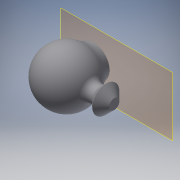
# Autodesk Inventor part: The Thing
Saved by Autodesk Inventor 2017 (Build 210142000, 142)
## iProperties
Created: 2017-03-09
Part Number: The Thing
Material: Generic
Document SubType Name: Modeling
Designer: PLTW
Density: 1 g/cm^3
Appearance: Default
Author: PLTW
Autodesk Inventor part; units mm, degrees
ref_plane "YZ Plane" through (0, 0, 0) normal (1, 0, 0) x (0, 1, 0)
ref_plane "XZ Plane" through (0, 0, 0) normal (0, 1, 0) x (-1, 0, 0)
sketch "Sketch3" plane through (0, 0, 0) normal (0, 0, 1) x (1, 0, 0)
  line L0 (-10.8841, 4.3559) -> (-10.16, 5.08)
  line L1 (-7.62, -2.54) -> (-10.16, -5.08)
  line L2 (-10.16, -5.08) -> (-10.8841, -4.3559)
  line L3 (-10.8912, 3.81) -> (-8.255, 6.4462)
  line L4 (-8.255, 6.4462) -> (-4.191, 2.3822)
  line L5 (-4.191, 2.3822) -> (-4.191, 0)
  line L6 (-4.191, 0) -> (-16.6062, 0)
  line L7 (-10.8912, 3.81) -> (-16.6062, 3.81)
  line L8 (-16.6062, 3.81) -> (-16.6062, 0)
  line L9 (-10.8841, 4.3559) -> (-9.525, 5.715)
  line L10 (-9.525, -5.715) -> (-10.8841, -4.3559)
  line L11 (-8.255, 6.985) -> (-3.81, 2.54)
  line L12 (-3.81, 2.54) -> (-3.81, -2.54)
  line L13 (-3.81, -2.54) -> (-8.255, -6.985)
  point P0 (0, 0)
  point P1 (-7.62, 0)
  dimension "d5" = 0.381
  dimension "d12" = 5.715
  dimension "d13" = 3.81
  dimension "d26" = 0.381
  dimension "d27" = 0.381
  constraints: 28 end point, 3 perpendicular, 2 horizontal alignment, 2 vertical, 1 horizontal, 1 parallel, 23 other
  measures "d5" distance between parallel lines of L0 L3
  measures "d12" distance of L3.start L7.end
  measures "d13" distance of L7.end L6.end
  measures "d26" distance between parallel lines of L11 L4
  measures "d27" distance between parallel lines of L12 L5
revolve "Revolution2" add sketch "Sketch3" angle 360 about axis through (-4.191, 0, 0) along (-1, 0, 0)
fillet "Fillet2" radius 0.127 3 edges at (-8.255, -6.4462, 0) (-10.8912, -3.81, 0) (-4.191, -2.3822, 0)
sketch "Sketch5" plane through (0, 0, 0) normal (0, 1, 0) x (-1, 0, 0)
  line L0 (16.6062, 3.81) -> (16.6062, -3.81) projected
  line L1 (16.6062, 3.81) -> (16.6062, -3.81) projected
  line L2 (10.9438, 3.81) -> (10.9438, -3.81) projected
  arc A0 (26.7662, 12.7) -> (26.7662, -12.7) centre (26.7662, 0) ccw
  line L3 (26.7662, 12.7) -> (26.7662, -12.7)
  point P0 (0, 0)
  dimension "d14" = 25.4
  dimension "d15" = 2.54
  constraints: 3 point on circle, 2 end point, 2 vertical alignment, 1 centre point, 1 horizontal alignment, 1 vertical
  measures "d14" distance of L3.end A0.start
  measures "d15" distance edge to line of A0 L0
revolve "Revolution3" add sketch "Sketch5" angle 360 about axis through (-26.7662, 0, 12.7) along (0, 0, -1)
ref_plane "Work Plane1" through (0, 0, -12.7) normal (0, 0, 1) x (1, 0, 0)
sketch "Sketch8" plane through (0, 0, -12.7) normal (0, 0, 1) x (1, 0, 0)
  line L0 (-14.6512, -3.81) -> (-14.6512, 3.81) projected
  arc A0 (-14.6512, 3.81) -> (-14.6512, -3.81) centre (-26.7662, 0) ccw projected
  circle A1 centre (-26.7662, 0) radius 7.62
  arc A2 (-6.8635, -3.3102) -> (-6.8635, 3.3102) centre (0, 0) ccw projected
  constraints: 1 centre point, 1 coincident, 1 equal radius
extrude "Extrusion1" add sketch "Sketch8" along normal up to next contours A1
fillet "Fillet3" radius 12.7 1 edges at (-34.3862, 0, -10.16)
fillet "Fillet4" radius 3.175 3 edges at (-14.6512, -3.81, 0) (-14.6512, 2.6939, 2.6943) (-14.6512, 2.6939, -2.6943)
equation "\"d26\" = d5"
equation "\"d27\" = d5"
body "Solid2"
